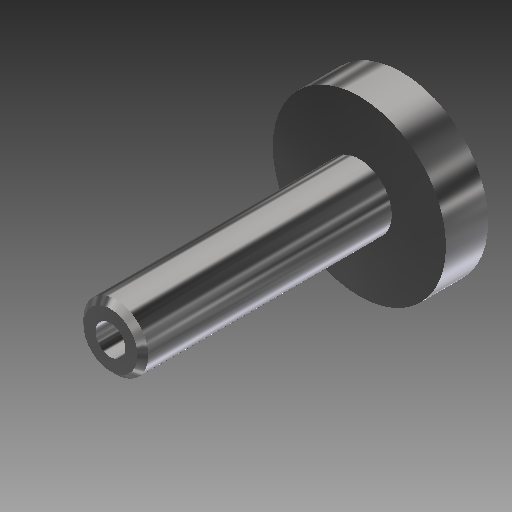
# Autodesk Inventor part: piston
Saved by Autodesk Inventor 2017 SP1 (Build 210196100, 196)
## iProperties
Created: 2017-06-14
Part Number: piston
Material: Stainless Steel
Document SubType Name: Modeling
Designer: RMcComber
Density: 1 g/cm^3
Appearance: Semi-Polished
Author: RMcComber
Autodesk Inventor part; units mm, degrees
ref_plane "YZ Plane" through (0, 0, 0) normal (1, 0, 0) x (0, 1, 0)
ref_plane "XZ Plane" through (0, 0, 0) normal (0, 1, 0) x (-1, 0, 0)
ref_plane "XY Plane" through (0, 0, 0) normal (0, 0, 1) x (1, 0, 0)
sketch "Sketch1" plane through (0, 0, 0) normal (0, 0, 1) x (1, 0, 0)
  circle A0 centre (0, 0) radius 16
  dimension "d0" = 32
  constraints: 1 centre point, 1 coincident
  measures "d0" diameter of A0
extrude "Extrusion1" add sketch "Sketch1" along normal blind 7.8
sketch "Sketch2" plane through (0, 0, 7.8) normal (0, 0, 1) x (1, 0, 0)
  circle A0 centre (0, 0) radius 16 projected
  circle A1 centre (0, 0) radius 6
  dimension "d3" = 12
  constraints: 1 centre point, 1 coincident
  measures "d3" diameter of A1
extrude "Extrusion2" add sketch "Sketch2" along normal blind 46 contours A1
sketch "Sketch3" plane through (0, 0, 53.8) normal (0, 0, 1) x (1, 0, 0)
  circle A0 centre (0, 0) radius 6 projected
  circle A1 centre (0, 0) radius 2.75
  dimension "d6" = 5.5
  constraints: 1 centre point, 1 coincident
  measures "d6" diameter of A1
extrude "Extrusion3" cut sketch "Sketch3" against normal blind 15 contours A1
chamfer "Chamfer1" distance 1 angle 45 1 edges at (-6, 0, 53.8)
body "Solid1"
